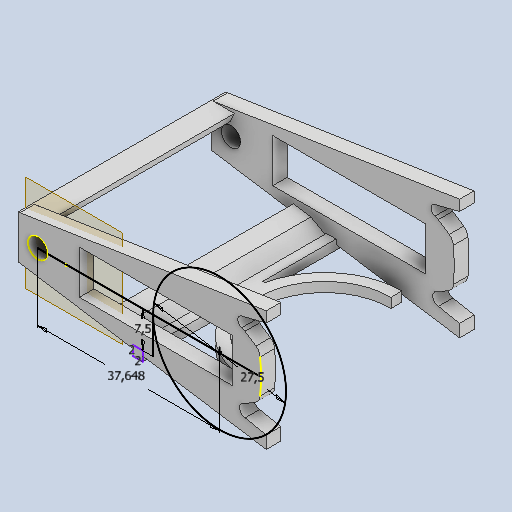
# Autodesk Inventor part: Cage
Saved by Autodesk Inventor 2025 (Build 290162000, 162)
## iProperties
Created: 2025-08-05
Part Number: Cage
Material: Generic
Document SubType Name: Modeling
Designer: Pravoslav
Density: 1 g/cm^3
Appearance: Default
Author: Pravoslav
Autodesk Inventor part; units mm, degrees
ref_plane "YZ Plane" through (0, 0, 0) normal (1, 0, 0) x (0, 1, 0)
ref_plane "XZ Plane" through (0, 0, 0) normal (0, 1, 0) x (-1, 0, 0)
ref_plane "Work Plane1" through (0, 0, 20) normal (0, 0, 1) x (1, 0, 0)
sketch "Sketch1" plane through (0, 0, 20) normal (0, 0, 1) x (1, 0, 0)
  circle A0 centre (-6, 0) radius 2
  line L0 (-10.0224, 4.5) -> (39.9776, 4.5)
  line L1 (39.9776, 4.5) -> (39.9776, -4.5)
  line L2 (39.9776, -4.5) -> (-10.0224, -4.5)
  line L3 (-10.0224, -4.5) -> (-10.0224, 4.5)
  line L4 (39.9776, 4.5) -> (36.5254, 6.8216)
  line L5 (39.9776, -4.5) -> (36.9512, -6.4067)
  arc A1 (36.5254, 9.0045) -> (36.5254, 6.8216) centre (36.4895, 7.9131) ccw
  arc A2 (36.9512, -6.4067) -> (36.9512, -8.9625) centre (37.0427, -7.6846) ccw
  line L6 (36.5254, 9.0045) -> (41.3206, 10.2245)
  line L7 (41.3206, 10.2245) -> (41.3206, 12.4243)
  line L8 (41.3206, 12.4243) -> (-9.6772, 4.5)
  line L9 (36.9512, -8.9625) -> (41.3206, -9.8433)
  line L10 (41.3206, -9.8433) -> (41.3206, -12.4334)
  line L11 (41.3206, -12.4334) -> (-10.0224, -4.5)
  circle A3 centre (-6, 0) radius 46.1973
  line L12 (2.6468, -4.5) -> (34.2776, -4.5)
  line L13 (34.2776, -4.5) -> (34.2776, 4.5)
  line L14 (34.2776, 4.5) -> (2.6468, 4.5)
  line L15 (2.6468, 4.5) -> (2.6468, -4.5)
  point P0 (0, 0)
  point P1 (2.6468, 4.5)
  dimension "d1" = 4
  dimension "d2" = 50
  dimension "d3" = 9
  dimension "d4" = 4.5
  dimension "d5" = 6
  constraints: 32 end point, 5 point on line, 4 parallel, 4 point on circle, 3 centre point, 2 horizontal, 2 perpendicular, 1 coincident, 1 vertical, 3 other
  measures "d1" diameter of A0
  measures "d2" distance of L1.end L2.end
  measures "d3" distance of L0.end L1.end
  measures "d4" distance from line of L0 point (0, 0)
  measures "d5" distance of point (0, 0) A0.centre
extrude "Extrusion1" add sketch "Sketch1" along normal mid plane 3 contours L0 L15 L2 L3 | L8 A3 L6 A1 L4 L0 | L2 L5 A2 L9 A3 L11 | L8 L7 L6 A3 | A3 L9 L10 L11 | L0 L1 L2 L13 | A3 L1
mirror "Mirror1" about plane through (0, 0, 0) normal (0, 0, 1) of "Extrusion1"
fillet "Fillet1" radius 2 8 edges at (39.9776, -4.5, -20) (39.9776, 4.5, -20) (39.9776, -4.5, 20) (39.9776, 4.5, 20) (36.5254, 6.8216, 20) (36.9512, -6.4067, 20) (36.9512, -6.4067, -20) (36.5254, 6.8216, -20)
sketch "Sketch2" plane through (-10.0224, -4.5, -18.5) normal (0, 0, 1) x (1, 0, 0)
  line L0 (0, 9) -> (0, 0) projected
  line L1 (10.0224, 7.1192) -> (0, 7.1192)
  line L2 (0, 7.1192) -> (0, 9)
  line L3 (0, 9) -> (10.0224, 9)
  line L4 (10.0224, 9) -> (10.0224, 7.1192)
  line L5 (0, 0) -> (51.3431, -7.9334) projected
  line L6 (24.3876, -3.7683) -> (16.7368, -2.5861)
  line L7 (16.9636, -1.0923) -> (24.6183, -2.2751)
  line L8 (24.6183, -2.2751) -> (24.3876, -3.7683)
  line L9 (16.7368, -2.5861) -> (16.9877, -0.9624)
  line L10 (16.9877, -0.9624) -> (16.7368, -2.5861)
  line L11 (24.3876, -3.7683) -> (16.7368, -2.5861)
  line L12 (3.8915, 7.1192) -> (4.7568, 9)
  line L13 (24.3876, -3.7683) -> (20.5622, -1.6484)
  point P0 (10.0224, 4.5)
  point P1 (16.9675, -1.0929)
  constraints: 24 end point, 5 point on line, 3 parallel, 2 collinear, 2 perpendicular, 1 horizontal
extrude "Extrusion2" add sketch "Sketch2" along normal up to surface (37 mm away) contours L3 L12 L1 L0 | L9 L7 L13 L5
sketch "Sketch3" plane through (0, 0, 21.5) normal (0, 0, 1) x (1, 0, 0)
  circle A0 centre (-6, 0) radius 2 projected
  line L0 (-6, 0) -> (40.1973, 0)
  arc A1 (40.0654, -3.4883) -> (40.0625, 3.5265) centre (-6, 0) ccw projected
  line L1 (-6, 0) -> (31.648, 0)
  line L2 (31.648, 0) -> (31.648, 1.0336)
  circle A2 centre (31.648, 0) radius 13.75
  line L3 (17.898, 0) -> (17.898, -7.5)
  line L4 (15.7607, -7.5) -> (13.7607, -7.5)
  line L5 (13.7607, -7.5) -> (13.7607, -9.5)
  line L6 (13.7607, -9.5) -> (15.7607, -9.5)
  line L7 (15.7607, -9.5) -> (15.7607, -7.5)
  point P0 (0, 0)
  dimension "d13" = 27.5
  dimension "d12" = 37.648
  dimension "d14" = 7.5
  dimension "d15" = 2
  dimension "d16" = 2
  constraints: 16 end point, 2 horizontal, 2 parallel, 2 perpendicular, 2 point on line, 2 vertical, 1 coincident, 1 horizontal alignment, 1 point on circle, 2 other
  measures "d12" distance of L0.start L1.end
  measures "d14" distance of L3.start L3.end
  measures "d15" distance of L6.end L5.end
  measures "d16" distance of L5.end L4.end
extrude "Extrusion3" add sketch "Sketch3" against normal up to surface (43 mm away) contours L7 L6 L5 L4
sketch "Sketch4" plane through (13.7607, -9.5, 21.5) normal (0, -1, 0) x (1, 0, 0)
  line L0 (18.1276, 0.5933) -> (18.1276, -42.6238)
  circle A0 centre (18.1276, -21.5) radius 13.75
  circle A1 centre (18.1276, -21.5) radius 16
  line L1 (2, -43) -> (27.56, -43) projected
  line L2 (0, -3) -> (0, -40) projected
  line L3 (0, -19.9291) -> (4.062, -19.9291)
  line L4 (4.062, -19.9291) -> (4.062, -24.7949)
  line L5 (4.062, -24.7949) -> (0, -24.7949)
  line L6 (0, -24.7949) -> (0, -19.9291)
  point P0 (-13.7607, -21.5)
  point P1 (2.4705, -24.7949)
  point P2 (18.1276, -37.5)
  point P3 (18.1276, -35.25)
  point P4 (18.1276, -7.75)
  point P5 (18.1276, -5.5)
  point P6 (2.2049, -19.9291)
  dimension "d19" = 27.5
  dimension "d20" = 32
  dimension "d21" = 21.5
  constraints: 10 end point, 2 centre point, 2 parallel, 2 point on line, 1 coincident, 1 horizontal, 1 perpendicular, 1 vertical
  measures "d19" diameter of A0
  measures "d20" diameter of A1
  measures "d21" distance from line of L1 A0.centre
extrude "Extrusion4" add sketch "Sketch4" against normal blind 2 contours L0 A0 A1 L5 L4 L3 | L3 L4 L5 A1 | A1 L5 L2 L3
body "Solid1"
